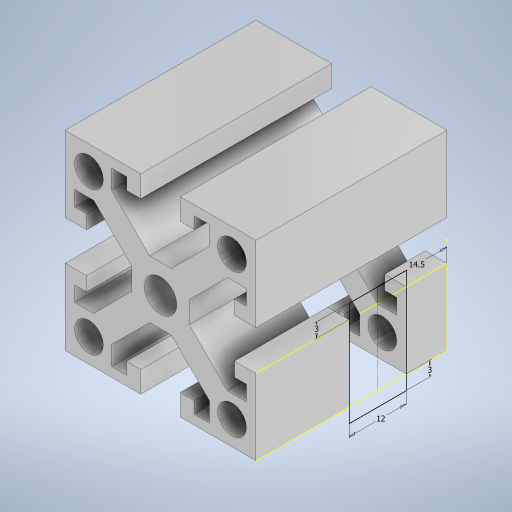
# Autodesk Inventor part: Aluminum_Profile_4040_40.10mm_left
Saved by Autodesk Inventor 2024.2 (Build 282272000, 272)
## iProperties
Created: 2023-08-26
Part Number: Aluminum_Profile_4040_40.10mm_left
Material: Aluminum 6061-AHC
Document SubType Name: Modeling
Designer: chanh
Density: 2.7 g/cm^3
Appearance: Aluminum - Dark
Author: chanh
Autodesk Inventor part; units mm, degrees
ref_plane "YZ Plane" through (0, 0, 0) normal (1, 0, 0) x (0, 1, 0)
ref_plane "XZ Plane" through (0, 0, 0) normal (0, 1, 0) x (-1, 0, 0)
ref_plane "XY Plane" through (0, 0, 0) normal (0, 0, 1) x (1, 0, 0)
sketch "Sketch1" plane through (0, 0, 0) normal (0, 0, 1) x (1, 0, 0)
  circle A0 centre (0, 0) radius 3.4
  line L0 (0, 0) -> (20, 20) construction
  line L1 (0, 0) -> (28.2843, 0) construction
  line L2 (20, 20) -> (4.15, 20)
  line L3 (4.15, 20) -> (4.15, 15.5)
  line L4 (4.15, 15.5) -> (7.1, 15.5)
  line L5 (7.1, 15.5) -> (7.1, 18)
  line L6 (7.1, 18) -> (10.25, 18)
  line L7 (10.25, 18) -> (10.25, 14)
  line L8 (0, 0) -> (0, 26.1056) construction
  line L9 (10.25, 14) -> (2.3, 6.05)
  line L10 (2.3, 6.05) -> (0, 6.05)
  circle A1 centre (15, 15) radius 3
  line L11 (20, 20) -> (20, 4.15)
  line L12 (20, 4.15) -> (15.5, 4.15)
  line L13 (15.5, 4.15) -> (15.5, 7.1)
  line L14 (15.5, 7.1) -> (18, 7.1)
  line L15 (18, 7.1) -> (18, 10.25)
  line L16 (18, 10.25) -> (14, 10.25)
  line L17 (14, 10.25) -> (6.05, 2.3)
  line L18 (6.05, 2.3) -> (6.05, 0)
  line L19 (-2.3, 6.05) -> (0, 6.05)
  line L20 (-10.25, 14) -> (-2.3, 6.05)
  line L21 (-10.25, 18) -> (-10.25, 14)
  line L22 (-4.15, 15.5) -> (-7.1, 15.5)
  line L23 (-7.1, 15.5) -> (-7.1, 18)
  line L24 (-7.1, 18) -> (-10.25, 18)
  line L25 (-4.15, 20) -> (-4.15, 15.5)
  line L26 (-20, 20) -> (-4.15, 20)
  circle A2 centre (-15, 15) radius 3
  line L27 (-20, 20) -> (-20, 4.15)
  line L28 (-14, 10.25) -> (-6.05, 2.3)
  line L29 (-18, 7.1) -> (-18, 10.25)
  line L30 (-18, 10.25) -> (-14, 10.25)
  line L31 (-20, 4.15) -> (-15.5, 4.15)
  line L32 (-15.5, 4.15) -> (-15.5, 7.1)
  line L33 (-15.5, 7.1) -> (-18, 7.1)
  line L34 (-6.05, 2.3) -> (-6.05, 0)
  line L35 (-6.05, -2.3) -> (-6.05, 0)
  line L36 (-14, -10.25) -> (-6.05, -2.3)
  line L37 (-18, -10.25) -> (-14, -10.25)
  line L38 (-15.5, -4.15) -> (-15.5, -7.1)
  line L39 (-15.5, -7.1) -> (-18, -7.1)
  line L40 (-18, -7.1) -> (-18, -10.25)
  line L41 (-20, -4.15) -> (-15.5, -4.15)
  line L42 (-20, -20) -> (-20, -4.15)
  circle A3 centre (-15, -15) radius 3
  line L43 (-20, -20) -> (-4.15, -20)
  line L44 (-10.25, -14) -> (-2.3, -6.05)
  line L45 (-7.1, -18) -> (-10.25, -18)
  line L46 (-10.25, -18) -> (-10.25, -14)
  line L47 (-4.15, -20) -> (-4.15, -15.5)
  line L48 (-4.15, -15.5) -> (-7.1, -15.5)
  line L49 (-7.1, -15.5) -> (-7.1, -18)
  line L50 (-2.3, -6.05) -> (0, -6.05)
  line L51 (2.3, -6.05) -> (0, -6.05)
  line L52 (10.25, -14) -> (2.3, -6.05)
  line L53 (10.25, -18) -> (10.25, -14)
  line L54 (4.15, -15.5) -> (7.1, -15.5)
  line L55 (7.1, -15.5) -> (7.1, -18)
  line L56 (7.1, -18) -> (10.25, -18)
  line L57 (4.15, -20) -> (4.15, -15.5)
  line L58 (20, -20) -> (4.15, -20)
  circle A4 centre (15, -15) radius 3
  line L59 (20, -20) -> (20, -4.15)
  line L60 (14, -10.25) -> (6.05, -2.3)
  line L61 (18, -7.1) -> (18, -10.25)
  line L62 (18, -10.25) -> (14, -10.25)
  line L63 (20, -4.15) -> (15.5, -4.15)
  line L64 (15.5, -4.15) -> (15.5, -7.1)
  line L65 (15.5, -7.1) -> (18, -7.1)
  line L66 (6.05, -2.3) -> (6.05, 0)
  point P0 (0, 6.05)
  point P1 (-6.05, 0)
  point P2 (0, -6.05)
  dimension "d0" = 6.8
  dimension "d1" = 45
  dimension "d2" = 20
  dimension "d3" = 6
  dimension "d4" = 15
  dimension "d5" = 10.25
  dimension "d6" = 7.1
  dimension "d7" = 4.15
  dimension "d8" = 4.5
  dimension "d9" = 2
  dimension "d10" = 13.95
  dimension "d11" = 6
  dimension "d14" = 360
  constraints: 134 end point, 8 symmetric about line, 5 centre point, 5 perpendicular, 2 horizontal, 2 point on line, 2 vertical, 1 coincident, 1 equal length, 1 parallel, 141 other
  measures "d0" diameter of A0
  measures "d1" angle of L1 L0
  measures "d2" horizontal distance of L0.end point (0, 0)
  measures "d3" diameter of A1
  measures "d4" horizontal distance of A1.centre point (0, 0)
  measures "d5" distance between parallel lines of L7 L8
  measures "d6" distance between parallel lines of L8 L5
  measures "d7" distance between parallel lines of L8 L3
  measures "d8" distance between parallel lines of L4 L2
  measures "d9" distance between parallel lines of L2 L6
  measures "d10" distance between parallel lines of L2 L10
  measures "d11" distance from line of L7.end L2
extrude "Extrusion1" add sketch "Sketch1" along normal blind 40
sketch "Sketch3" plane through (20, -20, 0) normal (1, 0, 0) x (0, 0, -1)
  line L0 (-14.5, 15.85) -> (-14.5, 0) construction
  line L1 (-20.5, 18.85) -> (-20.5, -3)
  line L2 (-8.5, 18.85) -> (-8.5, -3)
  line L3 (0, 15.85) -> (-40, 15.85) projected
  line L4 (0, 0) -> (-40, 0) projected
  line L5 (0, 0) -> (0, 15.85) projected
  line L6 (-20.5, 18.85) -> (-8.5, 18.85)
  line L7 (-20.5, -3) -> (-8.5, -3)
  point P0 (0, 20)
  dimension "d22" = 14.5
  dimension "d23" = 12
  dimension "d24" = 3
  dimension "d25" = 3
  constraints: 10 end point, 2 symmetric about line, 1 horizontal, 1 perpendicular, 2 other
  measures "d22" distance between parallel lines of L5 L0
  measures "d23" distance between parallel lines of L2 L1
  measures "d24" distance of the line from the sketch origin of L7
extrude "Extrusion3" cut sketch "Sketch3" against normal up to surface (13.95 mm away) contours L6 L2 L3 L1 | L3 L2 L4 L1 | L4 L2 L7 L1
body "Solid1"
